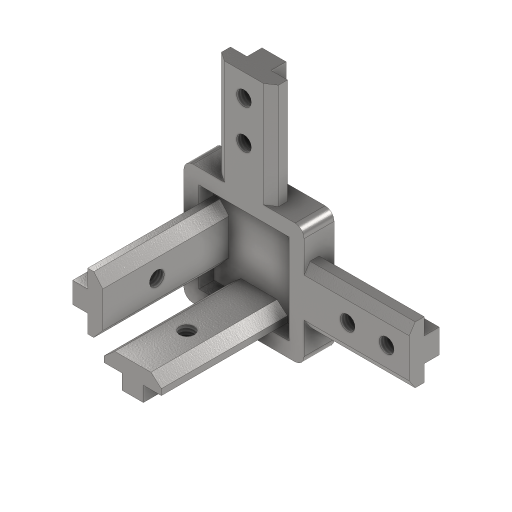
# Autodesk Inventor part: Sambungan Siku
Saved by Autodesk Inventor 2024.4 (Build 284460000, 460)
## iProperties
Created: 2025-10-20
Part Number: Sambungan Siku
Material: Generic
Document SubType Name: Modeling
Designer: Hp
Density: 1 g/cm^3
Appearance: Galvanized
Author: Hp
Autodesk Inventor part; units mm, degrees
ref_plane "YZ Plane" through (0, 0, 0) normal (1, 0, 0) x (0, 1, 0)
ref_plane "XZ Plane" through (0, 0, 0) normal (0, 1, 0) x (-1, 0, 0)
sketch "Sketch1" plane through (0, 0, 0) normal (0, 0, 1) x (1, 0, 0)
  line L0 (20, -20) -> (-20, -20)
  line L1 (-20, -20) -> (-20, 20)
  line L2 (-20, 20) -> (20, 20)
  line L3 (20, 20) -> (20, -20)
  line L4 (20, -20) -> (-20, 20) construction
  line L5 (-20, -20) -> (20, 20) construction
  point P0 (0, 0)
  dimension "d0" = 40
  dimension "d1" = 40
  constraints: 12 end point, 2 midpoint, 2 parallel, 1 horizontal, 1 perpendicular
  measures "d0" distance of L1.end L2.end
  measures "d1" distance of L2.end L0.start
extrude "Extrusion1" add sketch "Sketch1" along normal blind 10
shell "Shell1" thickness 5 removed faces 1 at (6.6667, -6.6667, 10)
sketch "Sketch2" plane through (-15, 15, 5) normal (0, 0, 1) x (1, 0, 0)
  line L0 (0, 0) -> (30, 0) construction
  line L1 (0, -30) -> (0, 0) construction
  line L2 (30, -30) -> (0, -30) construction
  line L3 (30, 0) -> (30, -30) construction
  line L4 (18.5, -35) -> (11.5, -35)
  line L5 (5.5, -30) -> (24.5, -30)
  line L6 (-5, -35) -> (35, -35) projected
  line L7 (5.5, -30) -> (5.5, -28)
  line L8 (5.5, -28) -> (9, -25)
  line L9 (9, -25) -> (21, -25)
  line L10 (21, -25) -> (24.5, -28)
  line L11 (24.5, -28) -> (24.5, -30)
  line L12 (11.5, -30) -> (11.5, -35)
  line L13 (18.5, -35) -> (18.5, -30)
  point P0 (15, -15)
  point P1 (15, -35)
  point P2 (15, -35)
  point P3 (15, -25)
  point P4 (15, -35)
  point P5 (15, -30)
  dimension "d6" = 12
  dimension "d7" = 7
  dimension "d9" = 19
  dimension "d10" = 5
  dimension "d11" = 2
  dimension "d26" = 9.5
  dimension "d27" = 49.399
  constraints: 18 end point, 5 midpoint, 5 point on line, 3 perpendicular, 2 horizontal, 2 parallel, 2 vertical alignment, 1 coincident, 1 collinear, 1 vertical
  measures "d6" distance of L8.end L9.end
  measures "d7" distance between parallel lines of L12 L13
  measures "d9" distance of L5.start L5.end
  measures "d10" distance between parallel lines of L5 L9
  measures "d11" distance of L10.end L5.end
  measures "d26" distance from line of point (15, -15) L11
  measures "d27" angle of L11 L10
extrude "Extrusion2" add sketch "Sketch2" along normal blind 42
sketch "Sketch3" plane through (-6, -10, 5) normal (0, 1, 0) x (1, 0, 0)
  circle A0 centre (6, -24) radius 2.5
  line L0 (12, -42) -> (0, -42) construction
  line L1 (26, -5) -> (-14, -5) construction
  point P0 (6, 5)
  point P1 (6, -42)
  dimension "d16" = 5
  dimension "d17" = 18
  dimension "d18" = 37
  constraints: 1 centre point, 1 midpoint, 1 vertical alignment
  measures "d16" diameter of A0
  measures "d17" distance from line of L0 A0.centre
  measures "d18" distance from line of L0.end L1
hole "Hole1" at (0, -10, 29) direction (0, -1, 0) diameter 4.917 end through all thread size "M6x1" class "6H" standard "ANSI Metric M Profile"
ref_plane "Work Plane1" through (-20, -20, 0) normal (-0.7071068, 0.7071068, 0) x (0, 0, -1)
mirror "Mirror1" about plane through (-20, -20, 0) normal (-0.7071068, 0.7071068, 0) of "Extrusion2", "Hole1"
sketch "Sketch4" plane through (-20, 20, 0) normal (0, 1, 0) x (1, 0, 0)
  line L0 (16, 0) -> (24, 0)
  line L1 (29.5, -5) -> (10.5, -5)
  line L2 (29.5, -5) -> (29.5, -8)
  line L3 (29.5, -8) -> (26.5, -10)
  line L4 (26.5, -10) -> (13.5, -10)
  line L5 (13.5, -10) -> (10.5, -8)
  line L6 (10.5, -8) -> (10.5, -5)
  line L7 (24, -5) -> (24, 0)
  line L8 (16, 0) -> (16, -5)
  line L9 (40, 0) -> (0, 0) construction
  line L10 (40, -10) -> (0, -10) construction
  point P0 (20, 0)
  point P1 (18.964, 16.737)
  point P2 (22.1197, 0)
  point P3 (20, 0)
  point P4 (20, -10)
  point P5 (20, 0)
  point P6 (20, -5)
  point P7 (20, -10)
  point P8 (20, 0)
  point P9 (20, 0)
  point P10 (20, -10)
  point P11 (20, 0)
  dimension "d28" = 13
  dimension "d29" = 8
  dimension "d30" = 19
  dimension "d31" = 5
  dimension "d32" = 3
  dimension "d33" = 8.464
  dimension "d34" = 56.31
  dimension "d37" = 0
  dimension "d38" = 16.737
  dimension "d39" = 7.3803
  dimension "d40" = 9.5
  constraints: 18 end point, 8 midpoint, 3 parallel, 3 point on line, 3 vertical alignment, 2 coincident, 2 equal length, 2 perpendicular
  measures "d28" distance of L4.start L5.start
  measures "d29" distance between parallel lines of L7 L8
  measures "d30" distance of L2.start L1.end
  measures "d31" distance between parallel lines of L1 L4
  measures "d32" distance of L5.end L1.end
  measures "d33" distance from line of point (18.964, 16.737) L6
  measures "d34" angle of L6 L5
  measures "d37" distance from line of point (20, 0) L9
  measures "d38" distance from line of point (18.964, 16.737) L9
  measures "d39" distance from line of point (22.12, 0) L2
  measures "d40" distance from line of point (20, 0) L2
extrude "Extrusion3" add sketch "Sketch4" along normal blind 35
sketch "Sketch5" plane through (0, 0, 10) normal (0, 0, 1) x (1, 0, 0)
  line L0 (0, 47.5) -> (0, 34.5) construction
  line L1 (-6.5, 55) -> (6.5, 55) construction
  point P0 (0, 0)
  point P1 (0, 55)
  dimension "d41" = 7.5
  dimension "d42" = 13
  constraints: 2 end point, 1 midpoint, 1 vertical, 1 vertical alignment
  measures "d41" distance from line of L1 L0.start
  measures "d42" distance of L0.start L0.end
hole "Hole2" at (0, 34.5, 10) at (0, 47.5, 10) direction (0, 0, -1) diameter 4.917 end through all thread size "M6x1" class "6H" standard "ANSI Metric M Profile"
mirror "Mirror2" about plane through (-20, -20, 0) normal (-0.7071068, 0.7071068, 0) of "Hole2", "Extrusion3"
sketch "Sketch6" plane through (-15, 15, 5) normal (0, 0, 1) x (1, 0, 0)
  line L0 (30, -30) -> (30, 0) projected
  line L1 (30, -1.3137) -> (28.6863, 0)
  line L2 (0, 0) -> (30, 0) projected
  line L3 (30, -8.3848) -> (21.6152, 0)
  line L4 (35, -11) -> (35, 5) projected
  line L5 (30, 0) -> (30, -30) projected
  point P0 (15, -15)
  point P1 (30, -8.3848)
  dimension "d50" = 5
  dimension "d51" = 13
  dimension "d52" = 45
  constraints: 4 end point, 4 point on line, 1 parallel
  measures "d50" distance between parallel lines of L1 L3
  measures "d51" distance from line of L4.end L3
  measures "d52" angle of L0 L1
extrude "Extrusion4" add sketch "Sketch6" along normal blind 1.5 contours L3 L2 L1 L0
chamfer "Chamfer1" distance 0.5 angle 45 2 edges at (10.8076, 10.8076, 6.5) (14.3431, 14.3431, 6.5)
fillet "Fillet1" radius 3 4 edges at (20, 20, 5) (-20, 20, 5) (-20, -20, 5) (20, -20, 5)
equation "\"d26\" = 0.5 * d9"
body "Solid1"
